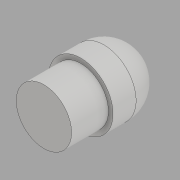
# Autodesk Inventor part: 2-2-3
Saved by Autodesk Inventor 2019 (Build 230136000, 136)
## iProperties
Created: 2020-11-06
Part Number: 2-2-3
Material: 一般
Document SubType Name: Modeling
Designer: Sugar
Density: 1 g/cm^3
Appearance: 預設
Author: Sugar
Autodesk Inventor part; units mm, degrees
ref_plane "YZ Plane" through (0, 0, 0) normal (1, 0, 0) x (0, 1, 0)
ref_plane "XZ Plane" through (0, 0, 0) normal (0, 1, 0) x (-1, 0, 0)
ref_plane "XY Plane" through (0, 0, 0) normal (0, 0, 1) x (1, 0, 0)
sketch "草圖1" plane through (0, 0, 0) normal (0, 0, 1) x (1, 0, 0)
  line L0 (-50, 0) -> (-50, -15)
  line L1 (-50, -15) -> (-30, -15)
  line L2 (-30, -15) -> (-30, -17.5)
  line L3 (-30, -17.5) -> (-17.5, -17.5)
  arc A0 (-17.5, -17.5) -> (0, 0) centre (-17.5, 0) ccw
  line L4 (0, 0) -> (-50, 0)
  dimension "d0" = 15
  dimension "d1" = 20
  dimension "d2" = 50
  dimension "d3" = 17.5
  constraints: 10 end point, 2 parallel, 2 point on circle, 2 vertical, 1 centre point, 1 coincident, 1 line through centre, 1 perpendicular, 1 tangent
  measures "d0" distance of L0.start L0.end
  measures "d1" distance of L0.end L1.end
  measures "d2" distance of L4.start L0.start
  measures "d3" radius of A0
revolve "迴轉1" add sketch "草圖1" angle 360 about axis through (0, 0, 0) along (-1, 0, 0)
